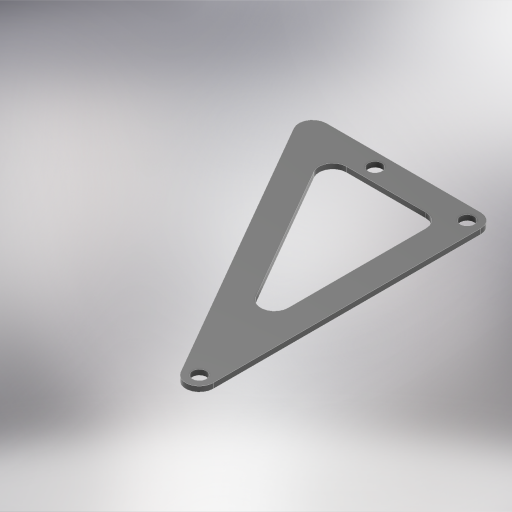
# Autodesk Inventor part: sheet1
Saved by Autodesk Inventor 2023 (Build 270158000, 158)
## iProperties
Created: 2023-03-30
Part Number: sheet1
Material: Acetal Resin, Black
Document SubType Name: Modeling
Designer: aaron
Density: 1.425 g/cm^3
Appearance: Smooth - Black
Author: aaron
Autodesk Inventor part; units mm, degrees
ref_plane "YZ Plane" through (0, 0, 0) normal (1, 0, 0) x (0, 1, 0)
ref_plane "XZ Plane" through (0, 0, 0) normal (0, 1, 0) x (-1, 0, 0)
ref_plane "XY Plane" through (0, 0, 0) normal (0, 0, 1) x (1, 0, 0)
sketch "Sketch2" plane through (0, 0, 0) normal (0, 1, 0) x (-1, 0, 0)
  circle A0 centre (0, 0) radius 34.925
  line L0 (0, 0) -> (0, -38.1)
  line L1 (0, -38.1) -> (-14.1986, -38.1)
  line L2 (-14.1986, -38.1) -> (14.1986, -38.1)
  circle A1 centre (14.1986, -38.1) radius 2.159
  circle A2 centre (-14.1986, -38.1) radius 2.159
  circle A3 centre (-14.1986, -38.1) radius 4.2333
  line L3 (-14.1986, -38.1) -> (-14.1986, 44.45) construction
  line L4 (-9.9653, -38.1) -> (-9.9653, 44.45)
  line L5 (-18.4319, 44.45) -> (-18.4319, -38.1)
  arc A4 (-18.4319, -38.1) -> (-9.9653, -38.1) centre (-14.1986, -38.1) ccw
  arc A5 (-9.9653, 44.45) -> (-18.4319, 44.45) centre (-14.1986, 44.45) ccw
  line L6 (-14.1986, 44.45) -> (33.4617, -38.1) construction
  line L7 (-17.8648, 42.3333) -> (29.7955, -40.2167)
  line L8 (37.1278, -35.9833) -> (-10.5324, 46.5667)
  arc A6 (-10.5324, 46.5667) -> (-17.8648, 42.3333) centre (-14.1986, 44.45) ccw
  arc A7 (29.7955, -40.2167) -> (37.1278, -35.9833) centre (33.4617, -38.1) ccw
  line L9 (-14.1986, 44.45) -> (81.1219, 44.45) construction
  line L10 (-14.1986, -38.1) -> (33.4617, -38.1) construction
  line L11 (-14.1986, -33.8667) -> (33.4617, -33.8667)
  line L12 (33.4617, -42.3333) -> (-14.1986, -42.3333)
  arc A8 (-14.1986, -33.8667) -> (-14.1986, -42.3333) centre (-14.1986, -38.1) ccw
  arc A9 (33.4617, -42.3333) -> (33.4617, -33.8667) centre (33.4617, -38.1) ccw
  point P0 (-14.1986, 3.175)
  point P1 (9.6315, 3.175)
  point P2 (9.6315, -38.1)
  point P3 (-9.9653, 28.651)
  point P4 (26.1293, -33.8667)
  point P5 (-9.9653, -33.8667)
  point P6 (-18.4319, -38.1)
  dimension "d17" = 69.85
  dimension "d18" = 38.1
  dimension "d19" = 14.1986
  dimension "d20" = 28.3972
  dimension "d21" = 4.318
  dimension "d22" = 4.318
  dimension "d23" = 8.4667
  dimension "d24" = 82.55
  dimension "d25" = 8.4667
  dimension "d26" = 60
  dimension "d27" = 8.4667
  constraints: 32 end point, 12 point on circle, 12 tangent, 10 centre point, 4 coincident, 3 midpoint, 3 parallel, 2 perpendicular, 2 vertical, 1 concentric, 1 equal length, 1 horizontal, 1 point on line
  measures "d17" diameter of A0
  measures "d18" distance of L0.start L0.end
  measures "d19" distance of L0.end L1.end
  measures "d20" distance of L1.end L2.end
  measures "d21" diameter of A1
  measures "d22" diameter of A2
  measures "d23" diameter of A3
  measures "d24" distance of L3.start L3.end
  measures "d25" diameter of A5
  measures "d26" angle of L6 L9
  measures "d27" diameter of A7
extrude "Extrusion2" add sketch "Sketch2" along normal blind 1.5875 contours L8 A0 L7 L4 | A0 L4 A5 L8 | L8 A9 L11 L7 A0 | L4 L7 A0 | A0 L7 A6 A5 L4 | A7 L7 L11 A9 | L7 L4 A0 L5 | A0 L5 A6 L7 | L11 L7 A7 L12 A3 L1 L0 A0 | A0 L0 L11 | L4 L11 A3 L5 A0 | L0 L1 L4 L11 A0 | A0 L11 L0 | A3 | L4 A3 L11
fillet "Fillet4" radius 4.2333 3 edges at (-26.1293, 0.7937, -33.8667) (9.9653, 0.7937, -33.8667) (9.9653, 0.7937, 28.651)
sketch "Sketch3" plane through (0, 1.5875, 0) normal (0, 1, 0) x (1, 0, 0)
  arc A0 (10.5324, -46.5667) -> (18.4319, -44.45) centre (14.1986, -44.45) ccw projected
  circle A1 centre (14.1986, -44.45) radius 2.159
  point P0 (0, 0)
  dimension "d31" = 4.318
  constraints: 1 centre point, 1 coincident
  measures "d31" diameter of A1
extrude "Extrusion3" cut sketch "Sketch3" against normal blind 1.5875
body "Solid2"
